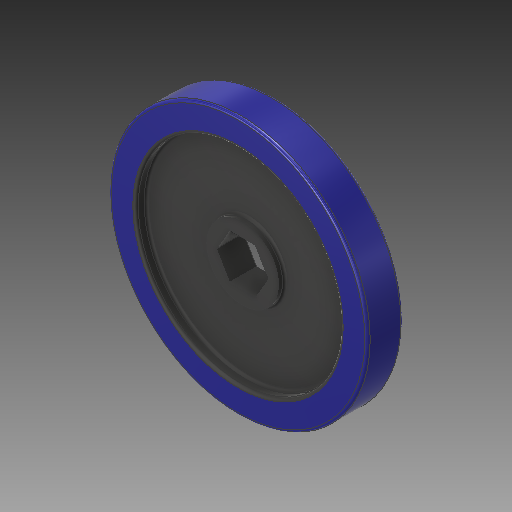
# Autodesk Inventor part: BaneBot 2 7-8 Blue
Saved by Autodesk Inventor 2017 (Build 210142000, 142)
## iProperties
Created: 2016-02-07
Part Number: BaneBot 2 7-8 Blue
Material: ABS Plastic
Document SubType Name: Modeling
Designer: FIRSTUser
Density: 1.06 g/cm^3
Appearance: Smooth - White
Author: FIRSTUser
Autodesk Inventor part; units mm, degrees
ref_plane "YZ Plane" through (0, 0, 0) normal (1, 0, 0) x (0, 1, 0)
ref_plane "XZ Plane" through (0, 0, 0) normal (0, 1, 0) x (-1, 0, 0)
ref_plane "XY Plane" through (0, 0, 0) normal (0, 0, 1) x (1, 0, 0)
sketch "Sketch1" plane through (0, 0, 0) normal (0, 0, 1) x (1, 0, 0)
  circle A0 centre (0, 0) radius 36.5125
  dimension "d0" = 73.025
  constraints: 1 centre point, 1 coincident
  measures "d0" diameter of A0
extrude "Extrusion1" add sketch "Sketch1" along normal mid plane 3.81
sketch "Sketch2" plane through (0, 0, 0) normal (0, 0, 1) x (1, 0, 0)
  circle A0 centre (0, 0) radius 36.5125 projected
  circle A1 centre (0, 0) radius 28.8925
  dimension "d3" = 57.785
  constraints: 1 centre point, 1 coincident
  measures "d3" diameter of A1
extrude "Extrusion2" add sketch "Sketch2" along normal mid plane 10.16
sketch "Sketch3" plane through (0, 0, 0) normal (0, 0, 1) x (1, 0, 0)
  circle A0 centre (0, 0) radius 10.16
  dimension "d6" = 20.32
  constraints: 1 centre point, 1 coincident
  measures "d6" diameter of A0
extrude "Extrusion3" add sketch "Sketch3" along normal mid plane 7.62
sketch "Sketch4" plane through (0, 0, 0) normal (0, 0, 1) x (1, 0, 0)
  line L0 (7.3323, 0) -> (3.6662, -6.35)
  line L1 (3.6662, -6.35) -> (-3.6662, -6.35)
  line L2 (-3.6662, -6.35) -> (-7.3323, 0)
  line L3 (-7.3323, 0) -> (-3.6662, 6.35)
  line L4 (-3.6662, 6.35) -> (3.6662, 6.35)
  line L5 (3.6662, 6.35) -> (7.3323, 0)
  point P0 (0, 0)
  point P1 (0, 0)
  dimension "d9" = 12.7
  constraints: 12 end point, 1 coincident, 13 other
  measures "d9" distance between parallel lines of L1 L4
extrude "Extrusion4" cut sketch "Sketch4" along normal mid plane 7.62
fillet "Fillet1" radius 0.762 8 edges at (-28.8925, 0, -5.08) (-28.8925, 0, 5.08) (-10.16, 0, 1.905) (-10.16, 0, -1.905) (-28.8925, 0, 1.905) (-28.8925, 0, -1.905) (-36.5125, 0, 5.08) (-36.5125, 0, -5.08)
body "Solid1"
